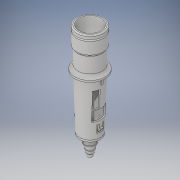
# Autodesk Inventor part: venturivalve
Saved by Autodesk Inventor 2019.1 (Build 231200000, 200)
## iProperties
Created: 2020-03-22
Part Number: venturivalve
Material: Generic
Document SubType Name: Modeling
Designer: rob
Density: 1 g/cm^3
Appearance: Default
Author: rob
## iProperties of the stored document venturivalve_3DPrint.ipt
Created: 2020-03-22
Part Number: venturivalve_3DPrint
Material: Generic
Document SubType Name: Modeling
Designer: Computus
Density: 1 g/cm^3
Appearance: Default
Author: Computus
Autodesk Inventor part; units mm, degrees
ref_plane "XZ Plane" through (0, 0, 0) normal (0, 1, 0) x (-1, 0, 0)
sketch "Sketch1" plane through (0, 0, 0) normal (0, 1, 0) x (-1, 0, 0)
  circle A0 centre (0, 0) radius 10.25
  circle A1 centre (0, 0) radius 9.3
  dimension "d0" = 20.5
  dimension "d1" = 18.6
  constraints: 2 centre point, 2 coincident
  measures "d0" diameter of A0
  measures "d1" diameter of A1
extrude "Extrusion1" add sketch "Sketch1" along normal blind 32
sketch "Sketch2" plane through (0, 32, 0) normal (0, 1, 0) x (1, 0, 0)
  circle A0 centre (0, 0) radius 11.25
  circle A1 centre (0, 0) radius 9.8591
  dimension "d4" = 22.5
  constraints: 2 centre point, 2 coincident
  measures "d4" diameter of A0
extrude "Extrusion2" add sketch "Sketch2" against normal blind 15.5
fillet "Fillet1" radius 1 1 edges at (-11.25, 32, 0)
ref_plane "Work Plane1" through (0, 28.7, 0) normal (0, 1, 0) x (1, 0, 0)
sketch "Sketch3" plane through (0, 28.7, 0) normal (0, 1, 0) x (1, 0, 0)
  circle A0 centre (0, 0) radius 10.25
  circle A1 centre (0, 0) radius 11.7527
  constraints: 2 centre point, 2 coincident
extrude "Extrusion3" cut sketch "Sketch3" against normal blind 0.3
fillet "Fillet2" radius 1 1 edges at (-11.25, 28.4, 0)
fillet "Fillet3" radius 1 2 edges at (-11.25, 16.5, 0) (10.25, 16.5, 0)
sketch "Sketch4" plane through (0, 0, 0) normal (0, -1, 0) x (1, 0, 0)
  circle A0 centre (0, 0) radius 12.75
  circle A1 centre (0, 0) radius 9.3
  dimension "d13" = 25.5
  constraints: 2 centre point, 2 coincident
  measures "d13" diameter of A0
extrude "Extrusion4" add sketch "Sketch4" along normal blind 1.5
fillet "Fillet4" radius 3 1 edges at (10.25, 0, 0)
sketch "Sketch5" plane through (0, 0, 0) normal (1, 0, 0) x (0, 1, 0)
  line L0 (-46.5, 8.75) -> (-46.5, 7.75)
  line L1 (0, -12.75) -> (0, 12.75) projected
  line L2 (-1.5, 12.75) -> (-1.5, -12.75) projected
  line L3 (-1.5, 10.25) -> (-46.5, 8.75)
  line L4 (-1.5, 9.25) -> (-46.5, 7.75)
  line L5 (-55.8, 0) -> (9.3, 0) projected
  point P0 (0, 0)
  constraints: 6 end point, 2 parallel, 2 point on line
revolve "Revolution1" add sketch "Sketch5" angle 360 about axis through (0, -10, 0) along (0, 1, 0)
sketch "Sketch6" plane through (0, -46.5, 0) normal (0, -1, 0) x (1, 0, 0)
  circle A0 centre (0, 0) radius 8.6832
  constraints: 1 centre point, 1 coincident
extrude "Extrusion5" add sketch "Sketch6" along normal blind 1.5
sketch "Sketch7" plane through (0, 0, 0) normal (1, 0, 0) x (0, 1, 0)
  line L0 (-48, 8.6832) -> (-48, -8.6832) projected
  line L1 (-48, 0) -> (-64, 0)
  line L2 (-48, 0) -> (-48, -4)
  line L3 (-64, 0) -> (-64, -2)
  line L4 (-61.6483, -2.6614) -> (-61.6483, -2)
  line L5 (-61.6483, -2) -> (-58.3066, -3.6013)
  line L6 (-58.3066, -3.6013) -> (-58.3066, -3.03)
  line L7 (-58.3066, -3.03) -> (-54.0121, -4.8091)
  line L8 (-54.0121, -4.2051) -> (-49.4337, -3.5968)
  line L9 (-54.0121, -4.2051) -> (-54.0121, -4.8091)
  line L10 (-64, -2) -> (-61.6483, -2.6614)
  line L11 (-49.4337, -3.5968) -> (-48, -4)
  line L12 (-76.8, 0) -> (12.8, 0) projected
  point P0 (0, 0)
  dimension "d21" = 16
  dimension "d22" = 4
  dimension "d23" = 2
  constraints: 22 end point, 2 vertical, 1 horizontal, 1 midpoint, 1 parallel, 1 perpendicular, 1 point on line
  measures "d21" distance of L1.start L1.end
  measures "d22" distance of L1.start L2.end
  measures "d23" distance of L1.end L3.end
revolve "Revolution2" add sketch "Sketch7" angle 360 about axis through (0, -10, 0) along (0, 1, 0)
sketch "Sketch8" plane through (0, -64, 0) normal (0, -1, 0) x (1, 0, 0)
  circle A0 centre (0, 0) radius 1.55
  dimension "d25" = 3.1
  constraints: 1 centre point, 1 coincident
  measures "d25" diameter of A0
sketch "Sketch9" plane through (0, -46.5, 0) normal (0, 1, 0) x (1, 0, 0)
  circle A0 centre (0, 0) radius 2.5
  dimension "d26" = 5
  constraints: 1 centre point, 1 coincident
  measures "d26" diameter of A0
extrude "Extrusion6" add sketch "Sketch9" along normal blind 32
fillet "Fillet5" radius 1.5 1 edges at (-2.5, -14.5, 0)
extrude "Extrusion7" cut sketch "Sketch8" against normal blind 70
ref_plane "Work Plane2" through (10, 0, 0) normal (1, 0, 0) x (0, 1, 0)
sketch "Sketch10" plane through (10, 0, 0) normal (1, 0, 0) x (0, 1, 0)
  line L0 (-42.3, -2.8) -> (-35.7, -2.8)
  line L1 (-35.7, 2.8) -> (-42.3, 2.8)
  line L2 (-42.3, 2.8) -> (-42.3, -2.8)
  line L3 (-48, 8.6832) -> (-48, -8.6832) projected
  line L4 (-57.6, 0) -> (9.6, 0) projected
  line L5 (-35.7, -1.2) -> (-41.3, -1.2)
  line L6 (-41.3, -1.2) -> (-41.3, 1.2)
  line L7 (-41.3, 1.2) -> (-35.7, 1.2)
  line L8 (-35.7, -2.8) -> (-35.7, -1.2)
  line L9 (-35.7, 1.2) -> (-35.7, 2.8)
  point P0 (0, 0)
  dimension "d34" = 5.6
  dimension "d35" = 5.7
  dimension "d36" = 2.8
  constraints: 16 end point, 4 parallel, 3 perpendicular, 2 horizontal
  measures "d34" distance of L1.start L0.end
  measures "d35" distance between parallel lines of L3 L2
  measures "d36" distance between parallel lines of L1 L4
extrude "Extrusion8" cut sketch "Sketch10" against normal blind 5
sketch "Sketch11" plane through (7.8319, -41.3, 1.2) normal (0, 0, 1) x (1, 0, 0)
  line L0 (1.0103, 0) -> (0, 0) projected
  line L1 (1.0103, 0) -> (1.0941, 2.5521)
  line L2 (1.0941, 2.5521) -> (2.6027, 2.5521)
  line L3 (2.6027, 2.5521) -> (1.0103, 0)
  point P0 (-7.8319, 41.3)
  constraints: 6 end point, 1 parallel
extrude "Extrusion9" add sketch "Sketch11" against normal blind 2.5
ref_plane "Work Plane3" through (-10, 0, 0) normal (1, 0, 0) x (0, 1, 0)
sketch "Sketch12" plane through (-10, 0, 0) normal (1, 0, 0) x (0, 1, 0)
  line L0 (-42.2, 2.9) -> (-35.4, 2.9)
  line L1 (-35.4, -2.9) -> (-42.2, -2.9)
  line L2 (-42.2, -2.9) -> (-42.2, 2.9)
  line L3 (-48, 8.6832) -> (-48, -8.6832) projected
  line L4 (-57.6, 0) -> (9.6, 0) projected
  line L5 (-41.3, 1.2) -> (-41.3, -1.2) projected
  line L6 (-41.3, 1.2) -> (-35.4, 1.2)
  line L7 (-35.4, -1.2) -> (-41.3, -1.2)
  line L8 (-41.3, -1.2) -> (-41.3, 1.2)
  line L9 (-35.4, 2.9) -> (-35.4, 1.2)
  line L10 (-35.4, -1.2) -> (-35.4, -2.9)
  point P0 (0, 0)
  dimension "d45" = 6.8
  dimension "d46" = 5.8
  dimension "d47" = 5.8
  dimension "d48" = 2.9
  constraints: 16 end point, 4 parallel, 2 horizontal, 2 perpendicular
  measures "d45" distance of L1.start L1.end
  measures "d46" distance of L0.end L1.start
  measures "d47" distance between parallel lines of L3 L2
  measures "d48" distance between parallel lines of L1 L4
extrude "Extrusion10" cut sketch "Sketch12" along normal blind 3
sketch "Sketch13" plane through (-7.8319, -41.3, -1.2) normal (0, 0, -1) x (-1, 0, 0)
  line L0 (1.0103, 0) -> (0, 0) projected
  line L1 (1.0103, 0) -> (1.0943, 2.5176)
  line L2 (0.9181, -5.2) -> (2.4181, 39.8) projected
  line L3 (1.0943, 2.5176) -> (2.6016, 2.5176)
  line L4 (1.0914, 0) -> (1.0103, 0) projected
  line L5 (2.6016, 2.5176) -> (1.0103, 0)
  point P0 (-7.8319, 41.3)
  constraints: 6 end point, 1 horizontal, 1 parallel
extrude "Extrusion11" add sketch "Sketch13" against normal blind 2.5 contours L1 L3 L2 L5 | L2 L3 L5
sketch "Sketch14" plane through (10, 0, 0) normal (1, 0, 0) x (0, 1, 0)
  line L0 (-33.2, -5.9) -> (-24.6, -5.9)
  line L1 (-24.6, -5.9) -> (-24.6, 5.9)
  line L2 (-24.6, 5.9) -> (-33.2, 5.9)
  line L3 (-33.2, 5.9) -> (-33.2, -5.9)
  line L4 (-42.84, 0) -> (7.14, 0) projected
  line L5 (-35.7, 1.2) -> (-35.7, 2.8) projected
  line L6 (-23.75, 5.9) -> (-9.95, 5.9)
  line L7 (-9.95, 5.9) -> (-9.95, 1.3)
  line L8 (-9.95, 1.3) -> (-23.75, 1.3)
  line L9 (-23.75, 1.3) -> (-23.75, 5.9)
  point P0 (0, 0)
  dimension "d53" = 8.6
  dimension "d54" = 11.8
  dimension "d55" = 5.9
  dimension "d56" = 2.5
  dimension "d57" = 13.8
  dimension "d58" = 4.6
  dimension "d59" = 0.85
  constraints: 16 end point, 4 parallel, 2 horizontal, 2 perpendicular, 1 point on line
  measures "d53" distance of L2.end L1.end
  measures "d54" distance of L1.end L0.end
  measures "d55" distance between parallel lines of L2 L4
  measures "d56" distance between parallel lines of L3 L5
  measures "d57" distance of L7.end L8.end
  measures "d58" distance of L6.end L7.end
  measures "d59" distance between parallel lines of L1 L9
extrude "Extrusion12" cut sketch "Sketch14" against normal blind 5
sketch "Sketch15" plane through (-10, 0, 0) normal (1, 0, 0) x (0, 1, 0)
  line L0 (-8.9, -6.7) -> (-22.7, -6.7)
  line L1 (-22.7, -6.7) -> (-22.7, -1.9)
  line L2 (-22.7, -1.9) -> (-8.9, -1.9)
  line L3 (-8.9, -1.9) -> (-8.9, -6.7)
  line L4 (-1.5, 12.75) -> (-1.5, -12.75) projected
  line L5 (-42.2, -2.9) -> (-35.4, -2.9) projected
  line L6 (-34.1141, -2.1509) -> (-31.4141, -2.1509)
  line L7 (-31.4141, -2.1509) -> (-31.4141, 2.6491)
  line L8 (-34.1141, 2.6491) -> (-34.1141, -2.1509)
  line L9 (-34.1141, 2.6491) -> (-34.1141, 7.6491)
  line L10 (-34.1141, 7.6491) -> (-31.4141, 2.6491)
  point P0 (0, 0)
  dimension "d62" = 13.8
  dimension "d63" = 4.8
  dimension "d64" = 7.4
  dimension "d65" = 1
  constraints: 18 end point, 3 parallel, 2 horizontal, 2 perpendicular, 1 vertical
  measures "d62" distance of L1.end L2.end
  measures "d63" distance of L0.end L1.end
  measures "d64" distance between parallel lines of L3 L4
  measures "d65" distance between parallel lines of L2 L5
extrude "Extrusion13" cut sketch "Sketch15" along normal blind 5
sketch "Sketch16" plane through (0, 0, 0) normal (1, 0, 0) x (0, 1, 0)
  arc A0 (-16, -2.5) -> (-14.5, -1) centre (-16, -1) ccw projected
  line L0 (-14.5478, -1.3755) -> (-10.9997, -8.9333)
  line L1 (-1.5, -9.25) -> (-46.5, -7.75) projected
  line L2 (-19.2614, -8.6804) -> (-25.0997, -2.5)
  line L3 (-46.5, -2.5) -> (-16, -2.5) projected
  line L4 (-25.0997, -2.5) -> (-14.5478, -1.3755)
  line L5 (-19.2614, -8.6804) -> (-10.9997, -8.9333)
  arc A1 (-14.5, 1) -> (-16, 2.5) centre (-16, 1) ccw projected
  line L6 (-1.5, 9.25) -> (-46.5, 7.75) projected
  line L7 (-46.5, 2.5) -> (-16, 2.5) projected
  line L8 (-14.5, 1) -> (-10.452, 8.9516)
  line L9 (-1.5, 9.25) -> (-46.5, 7.75) projected
  line L10 (-1.5, 9.25) -> (-46.5, 7.75) projected
  line L11 (-24, 8.5) -> (-10.452, 8.9516)
  line L12 (-1.5, 9.25) -> (-46.5, 7.75) projected
  line L13 (-24, 8.5) -> (-25.0997, 2.0607)
  arc A2 (-14.5, 1) -> (-16, 2.5) centre (-16, 1) ccw projected
  line L14 (-25.0997, 2.0607) -> (-14.5, 1)
  point P0 (0, 0)
  point P1 (-25.6325, 2.5)
  point P2 (-14.654, 2.5)
  constraints: 16 end point, 4 point on line, 1 collinear, 1 midpoint, 1 point on circle
extrude "Extrusion15" add sketch "Sketch16" along normal mid plane 2 contours A0 L0 L1 L2 L3 | L5 L2 L1 | L14 L13 L7 A1 | A1 L7 L13 L6 L8
sketch "Sketch17" plane through (10, 0, 0) normal (1, 0, 0) x (0, 1, 0)
  line L0 (-1.5, -9.25) -> (-1.5, 9.25) projected
  line L1 (-1.5, -0.7546) -> (-6.5, -0.7546)
  line L2 (-7, -0.2546) -> (-7, 0.5454)
  line L3 (-6.5, 1.0454) -> (-1.5, 1.0454)
  line L4 (-1.5, 1.0454) -> (-1.5, -0.7546)
  arc A0 (-7, -0.2546) -> (-6.5, -0.7546) centre (-6.5, -0.2546) ccw
  arc A1 (-6.5, 1.0454) -> (-7, 0.5454) centre (-6.5, 0.5454) ccw
  point P0 (0, 0)
  point P1 (-7, 1.0454)
  point P2 (-7, -0.7546)
  dimension "d75" = 5.5
  dimension "d76" = 1.8
  dimension "d77" = 0.5
  constraints: 8 end point, 4 point on circle, 4 point on line, 4 tangent, 2 centre point, 2 parallel, 1 equal radius, 1 horizontal, 1 perpendicular
  measures "d75" distance of point (-7, 1.045) L3.end
  measures "d76" distance of point (-7, -0.755) point (-7, 1.045)
  measures "d77" radius of A0
extrude "Extrusion16" add sketch "Sketch17" along normal blind 0.5
fillet "Fillet6" radius 3 2 edges at (0, -46.5, -7.75) (-2.5, -46.5, 0)
sketch "Sketch18" plane through (0, -64, 0) normal (0, -1, 0) x (1, 0, 0)
  circle A0 centre (0, 0) radius 1.55
  dimension "d83" = 3.1
  constraints: 1 centre point, 1 coincident
  measures "d83" diameter of A0
extrude "Extrusion17" cut sketch "Sketch18" against normal blind 50
body "Solid1"
